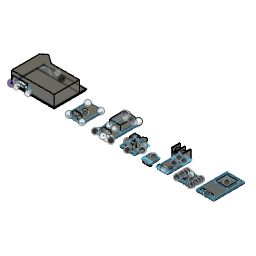
3D Module (Autodesk Fusion 360 design; units mm, degrees)
Autodesk Fusion 360 part; units mm, degrees
note: some values were not read from the file. Set by a fixed rule: which sketch regions a step uses.
sketch "Sketch3" plane through (0, 0, 0) normal (0, 0, 1) x (1, 0, 0)
sketch "LUX" plane through (0, 0, 0) normal (0, 0, 1) x (1, 0, 0)
  line L0 (77.07, 0) -> (94.93, 0)
  line L1 (97, 2.07) -> (97, 27.93)
  line L2 (94.93, 30) -> (77.07, 30)
  line L3 (75, 27.93) -> (75, 2.07)
  line L4 (86, 0) -> (86, 30) construction
  line L5 (86, 0) -> (91, 0) construction
  line L6 (91, 0) -> (91, 6) construction
  line L7 (91, 6) -> (86, 6) construction
  line L8 (86, 6) -> (86, 0) construction
  line L9 (91, 6) -> (81, 6)
  line L10 (81, 6) -> (81, 0)
  line L11 (81, 0) -> (91, 0)
  line L12 (91, 0) -> (91, 6)
  arc A0 (77.07, 30) -> (75, 27.93) centre (77.07, 27.93) ccw
  arc A1 (97, 27.93) -> (94.93, 30) centre (94.93, 27.93) ccw
  arc A2 (75, 2.07) -> (77.07, 0) centre (77.07, 2.07) ccw
  arc A3 (94.93, 0) -> (97, 2.07) centre (94.93, 2.07) ccw
  circle A4 centre (86, 15) radius 2.5
  dimension "d32" = 2.07
  constraint horizontal L0
  constraint vertical L1
  constraint horizontal L2
  constraint vertical L3
  constraint horizontal L5
  constraint vertical L6
  constraint horizontal L7
  constraint vertical L8
  constraint horizontal L9
  constraint vertical L10
  constraint horizontal L11
  constraint vertical L12
  constraint coincident L2 L4.end
  constraint tangent L2 A0
  constraint tangent L3 A0
  constraint tangent L1 A1
  constraint tangent L2 A1
  constraint equal A0 A1
  constraint coincident L0 L4.start
  constraint tangent L3 A2
  constraint tangent L0 A2
  constraint equal A0 A2
  constraint tangent L1 A3
  constraint tangent L0 A3
  constraint equal A0 A3
  constraint midpoint L4 A4.centre
  measures "d32" radius of A0
sketch "DHT" plane through (0, 0, 0) normal (0, 0, 1) x (1, 0, 0)
  line L0 (117.7, 0) -> (134.3, 0)
  line L1 (137, 2.7) -> (137, 38.8)
  line L2 (134.3, 41.5) -> (117.7, 41.5)
  line L3 (115, 38.8) -> (115, 2.7)
  arc A0 (117.7, 41.5) -> (115, 38.8) centre (117.7, 38.8) ccw
  arc A1 (137, 38.8) -> (134.3, 41.5) centre (134.3, 38.8) ccw
  arc A2 (115, 2.7) -> (117.7, 0) centre (117.7, 2.7) ccw
  arc A3 (134.3, 0) -> (137, 2.7) centre (134.3, 2.7) ccw
  line L4 (126, 6) -> (131, 6) construction
  line L5 (131, 0) -> (126, 0) construction
  line L6 (131, 6) -> (121, 6)
  line L7 (121, 6) -> (121, 0)
  line L8 (121, 0) -> (131, 0)
  line L9 (131, 0) -> (131, 6)
  line L10 (126, 41.5) -> (133.5, 41.5) construction
  line L11 (133.5, 16.5) -> (126, 16.5) construction
  line L12 (133.5, 16.5) -> (118.5, 16.5)
  line L13 (118.5, 41.5) -> (133.5, 41.5)
  line L14 (133.5, 16.5) -> (118.5, 16.5)
  line L15 (118.5, 16.5) -> (118.5, 36.5)
  line L16 (118.5, 36.5) -> (133.5, 36.5)
  line L17 (133.5, 36.5) -> (133.5, 16.5)
  line L18 (126, 41.5) -> (126, 36.5) construction
  line L19 (131.25, 36.5) -> (120.75, 36.5) construction
  line L20 (120.75, 41.5) -> (131.25, 41.5) construction
  line L21 (118.5, 36.5) -> (120.75, 41.5)
  line L22 (131.25, 41.5) -> (133.5, 36.5)
  circle A4 centre (126, 39) radius 1.75
  point P0 (115, 0)
  point P1 (137, 0)
  point P2 (115, 41.5)
  point P3 (126, 39)
  dimension "d25" = 22
  dimension "d26" = 41.5
  dimension "d63" = 2.7
  dimension "d65" = 10
  dimension "d66" = 6
  dimension "d68" = 25
  dimension "d69" = 15
  dimension "d70" = 20
  dimension "d71" = 10.5
  dimension "d72" = 3.5
  constraint horizontal L0
  constraint vertical L1
  constraint horizontal L2
  constraint vertical L3
  constraint coincident P2 L3
  constraint coincident P2 L2
  constraint tangent L3 A0
  constraint tangent L2 A0
  constraint tangent L1 A1
  constraint tangent L2 A1
  constraint equal A0 A1
  constraint coincident P0 L3
  constraint coincident P0 L0
  constraint tangent L3 A2
  constraint tangent L0 A2
  constraint equal A0 A2
  constraint coincident P1 L1
  constraint coincident P1 L0
  constraint tangent L1 A3
  constraint tangent L0 A3
  constraint equal A0 A3
  constraint midpoint L2 L10.start
  constraint horizontal L4
  constraint horizontal L5
  constraint horizontal L6
  constraint vertical L7
  constraint horizontal L8
  constraint vertical L9
  constraint horizontal L10
  constraint horizontal L11
  constraint horizontal L12
  constraint horizontal L13
  constraint horizontal L14
  constraint vertical L15
  constraint horizontal L16
  constraint vertical L17
  constraint midpoint L16 L18.end
  constraint horizontal L19
  constraint parallel L19 L20
  constraint midpoint L18 P3
  constraint coincident P3 A4.centre
  measures "d25" distance of P0 P1
  measures "d26" distance of P0 P2
  measures "d63" radius of A0
  measures "d65" distance of L4.end L6.end
  measures "d66" distance of L6 L8
  measures "d68" distance of L10.start L11.end
  measures "d69" distance of L11.start L12.end
  measures "d70" distance of L11.start L16.end
  measures "d71" distance of L20.start L20.end
  measures "d72" diameter of A4
sketch "DSM" plane through (0, 0, 0) normal (0, 0, 1) x (1, 0, 0) in component "DSM"
  line L0 (0, 0) -> (58.5, 0)
  line L1 (58.5, 0) -> (58.5, 35)
  line L2 (58.5, 35) -> (0, 35)
  line L3 (0, 35) -> (0, 0)
  line L4 (0, 0) -> (58.5, 0)
  line L5 (58.5, 0) -> (58.5, 44)
  line L6 (58.5, 44) -> (0, 44)
  line L7 (0, 44) -> (0, 0)
  line L8 (0, 35) -> (19.5, 35) construction
  line L9 (19.5, 44) -> (0, 44) construction
  line L10 (0, 44) -> (0, 35) construction
  line L11 (0, 44) -> (7, 44) construction
  line L12 (7, 0) -> (0, 0) construction
  line L13 (0, 0) -> (0, 44) construction
  line L14 (7, 44) -> (19.5, 35)
  line L15 (7, 44) -> (0, 38.3431)
  line L16 (29.25, 44) -> (29.25, 35) construction
  circle A0 centre (29.25, 39.5) radius 2
  line L17 (5.5, 0) -> (17.5, 0)
  line L18 (17.5, 0) -> (17.5, 5)
  line L19 (17.5, 5) -> (5.5, 5)
  line L20 (5.5, 5) -> (5.5, 0)
  line L21 (0, 0) -> (23, 0)
  line L22 (0, 5) -> (0, 0)
  line L23 (17.5, 5) -> (22, 5)
  line L24 (22, 5) -> (22, 0)
  line L25 (22, 0) -> (17.5, 0) construction
  line L26 (17.5, 0) -> (17.5, 5) construction
  line L27 (5.5, 5) -> (1, 5)
  line L28 (1, 5) -> (1, 0)
  line L29 (1, 0) -> (5.5, 0) construction
  line L30 (5.5, 0) -> (5.5, 5) construction
  dimension "d1" = 58.5
  dimension "d2" = 35
  dimension "d3" = 44
  dimension "d7" = 4
  constraint horizontal L0
  constraint vertical L1
  constraint horizontal L2
  constraint vertical L3
  constraint coincident L0.start L3.end
  constraint horizontal L4
  constraint vertical L5
  constraint horizontal L6
  constraint vertical L7
  constraint horizontal L8
  constraint horizontal L9
  constraint vertical L10
  constraint horizontal L11
  constraint horizontal L12
  constraint vertical L13
  constraint coincident L10 L15.end
  constraint equal L5 L13
  constraint midpoint L6 L16.start
  constraint midpoint L2 L16.end
  constraint midpoint L16 A0.centre
  constraint horizontal L17
  constraint vertical L18
  constraint horizontal L19
  constraint vertical L20
  constraint coincident L12 L17.start
  constraint horizontal L21
  constraint vertical L22
  constraint horizontal L23
  constraint vertical L24
  constraint horizontal L25
  constraint vertical L26
  constraint horizontal L27
  constraint vertical L28
  constraint horizontal L29
  constraint vertical L30
  measures "d1" distance of L0.start L0.end
  measures "d2" distance of L0.start L2.end
  measures "d3" distance of L0.start L6.end
  measures "d7" diameter of A0
extrude "Extrude7" add sketch "DSM" along normal blind 15.5 contours L0 L1 L2 L3 L4 L5 L7 L19 L21 L22 L23 L24 L27 L28 | L0 L4 L20 L21 L27 L28 | L0 L4 L17 L18 L19 L20 L21 | L2 L7 L14 L15 | L0 L4 L18 L21 L23 L24 makes body 1 in component "DSM"
extrude "Extrude4" cut sketch "DSM" along normal blind 10 contours L0 L4 L20 L21 L27 L28 | L0 L4 L17 L18 L19 L20 L21 | L0 L4 L18 L21 L23 L24 bodies 1 in component "DSM"
extrude "Extrude5" add sketch "DSM" against normal blind 1.5 bodies 1 in component "DSM"
extrude "Extrude8" add sketch "DSM" along normal blind 5 separate body contours L0 L4 L17 L18 L19 L20 L21 makes body 2
shell "Shell2" thickness 0.5 removed faces 1 at (9.5, 0, 1.6667) on bodies 2
copy_body "CutPasteBodies1" bodies 2 removing the originals makes body 3 in component "DSM"
extrude "Extrude9" add sketch "LUX" along normal blind 3 separate body contours A4 makes body 4
extrude "Extrude11" add sketch "LUX" against normal blind 1 contours L0 L1 L2 L3 L9 L10 L12 A0 A1 A2 A3 | L0 L9 L10 L11 L12 | A4 bodies 4
copy_body "Body->Comp1" bodies 4 removing the originals makes body 5 in component "LUX"
extrude "Extrude12" add sketch "LUX" along normal blind 5.5 separate body contours L0 L9 L10 L11 L12 makes body 6
shell "Shell4" thickness 0.5 removed faces 1 at (84.3333, 0, 3.6667) on bodies 6
copy_body "CutPasteBodies1'" bodies 6 removing the originals makes body 7 in component "LUX"
extrude "Extrude13" add sketch "DHT" along normal blind 8 separate body contours L12 L14 L15 L16 L17 makes body 8
extrude "Extrude14" add sketch "DHT" along normal blind 1.5 contours L2 L13 L16 L21 L22 bodies 8
extrude "Extrude15" add sketch "DHT" against normal blind 1 contours L0 L1 L2 L3 A0 A1 A2 A3 L6 L7 L9 L12 L13 L14 L15 L17 L21 L22 | L0 L6 L7 L8 L9 bodies 8
copy_body "Body->Comp2" bodies 8 removing the originals makes body 9 in component "DHT22"
extrude "Extrude16" add sketch "DHT" along normal blind 5.5 separate body contours L0 L6 L7 L8 L9 makes body 10
shell "Shell5" thickness 0.5 removed faces 1 at (124.3333, 0, 3.6667) on bodies 10
copy_body "CutPasteBodies1''" bodies 10 removing the originals makes body 11 in component "DHT22"
sketch "WSP" plane through (0, 0, 0) normal (0, 0, 1) x (1, 0, 0)
  line L0 (150, 0) -> (170, 0)
  line L1 (170, 0) -> (170, 20)
  line L2 (170, 20) -> (150, 20)
  line L3 (150, 20) -> (150, 0)
  line L4 (160, 20) -> (160, 0) construction
  circle A0 centre (150, 10) radius 2
  circle A1 centre (170, 10) radius 2
  circle A2 centre (160, 20) radius 2
  circle A3 centre (160, 0) radius 2
  circle A4 centre (150, 10) radius 1
  circle A5 centre (170, 10) radius 1
  line L5 (160, 2) -> (165, 2) construction
  line L6 (165, 2) -> (165, 7) construction
  line L7 (165, 7) -> (160, 7) construction
  line L8 (160, 7) -> (160, 2) construction
  line L9 (165, 7) -> (155, 7)
  line L10 (155, 7) -> (155, 2)
  line L11 (155, 2) -> (165, 2)
  line L12 (165, 2) -> (165, 7)
  line L13 (150, 20) -> (157, 20)
  line L14 (157, 20) -> (157, 13)
  line L15 (157, 13) -> (150, 13)
  line L16 (150, 13) -> (150, 20)
  circle A6 centre (166, 16) radius 4
  dimension "d82" = 20
  dimension "d83" = 20
  dimension "d84" = 4
  dimension "d85" = 4
  dimension "d86" = 4
  dimension "d87" = 4
  dimension "d88" = 2
  dimension "d89" = 2
  dimension "d91" = 5
  dimension "d92" = 10
  dimension "d93" = 7
  dimension "d94" = 7
  dimension "d95" = 4
  constraint horizontal L0
  constraint vertical L1
  constraint horizontal L2
  constraint vertical L3
  constraint midpoint L2 L4.start
  constraint midpoint L0 L4.end
  constraint midpoint L3 A0.centre
  constraint midpoint L1 A1.centre
  constraint coincident L4.start A2.centre
  constraint coincident L4.end A3.centre
  constraint concentric A0 A4
  constraint concentric A1 A5
  constraint horizontal L5
  constraint vertical L6
  constraint horizontal L7
  constraint vertical L8
  constraint coincident A3 L5.start
  constraint coincident L4 L5.start
  constraint horizontal L9
  constraint vertical L10
  constraint horizontal L11
  constraint vertical L12
  constraint horizontal L13
  constraint vertical L14
  constraint horizontal L15
  constraint vertical L16
  constraint tangent L2 A6
  constraint tangent L1 A6
  measures "d82" distance of L0.start L0.end
  measures "d83" distance of L0.start L2.end
  measures "d84" diameter of A0
  measures "d85" diameter of A1
  measures "d86" diameter of A2
  measures "d87" diameter of A3
  measures "d88" diameter of A4
  measures "d89" diameter of A5
  measures "d91" distance of L5.start L7.end
  measures "d92" distance of L6.end L9.end
  measures "d93" distance of L2.end L13.end
  measures "d94" distance of L2.end L15.end
  measures "d95" radius of A6
extrude "Extrude17" add sketch "WSP" along normal blind 5 separate body contours L2 L3 L13 L14 L15 L16 makes body 12
extrude "Extrude18" add sketch "WSP" along normal blind 7.5 separate body contours A6 makes body 13
extrude "Extrude19" add sketch "WSP" against normal blind 1.5 contours L9 L10 L11 L12 | L0 L1 L2 L3 A0 A1 A2 A3 L14 L15 A6 | L1 A1 A5 | L1 A1 A5 | L3 A0 A4 | L3 A0 A4 bodies 12 13
copy_body "Body->Comp3" bodies 12 removing the originals makes body 14 in component "WSP_bdy"
extrude "Extrude20" add sketch "WSP" along normal blind 8 separate body contours L9 L10 L11 L12 makes body 15
shell "Shell6" thickness 0.5 removed faces 1 at (160, 5.3333, 8) on bodies 15
copy_body "CutPasteBodies1'''" bodies 15 removing the originals makes body 16 in component "WSP_bdy"
sketch "SGP30" plane through (0, 0, 0) normal (0, 0, 1) x (1, 0, 0)
  line L0 (180, 0) -> (192, 0)
  line L1 (192, 0) -> (192, 12)
  line L2 (192, 12) -> (180, 12)
  line L3 (180, 12) -> (180, 0)
  line L4 (186, 12) -> (186, 0) construction
  line L5 (187.25, 8.7246) -> (184.75, 8.7246)
  line L6 (184.75, 8.7246) -> (184.75, 11.2246)
  line L7 (184.75, 11.2246) -> (187.25, 11.2246)
  line L8 (187.25, 11.2246) -> (187.25, 8.7246)
  line L9 (187.25, 8.7246) -> (184.75, 11.2246) construction
  line L10 (184.75, 8.7246) -> (187.25, 11.2246) construction
  line L11 (186, 0) -> (191, 0) construction
  line L12 (191, 0) -> (191, 2.45) construction
  line L13 (191, 2.45) -> (186, 2.45) construction
  line L14 (186, 2.45) -> (186, 0) construction
  line L15 (191, 2.45) -> (181, 2.45)
  line L16 (181, 2.45) -> (181, 0)
  line L17 (181, 0) -> (191, 0)
  line L18 (191, 0) -> (191, 2.45)
  point P0 (186, 9.9746)
  dimension "d105" = 12
  dimension "d106" = 12
  dimension "d107" = 2.5
  dimension "d108" = 2.5
  dimension "d110" = 2.45
  dimension "d111" = 10
  constraint horizontal L0
  constraint vertical L1
  constraint horizontal L2
  constraint vertical L3
  constraint midpoint L2 L4.start
  constraint midpoint L0 L4.end
  constraint horizontal L5
  constraint perpendicular L5 L6
  constraint parallel L5 L7
  constraint parallel L6 L8
  constraint coincident L9 P0
  constraint coincident L10 P0
  constraint coincident L4 P0
  constraint horizontal L11
  constraint vertical L12
  constraint horizontal L13
  constraint vertical L14
  constraint horizontal L15
  constraint vertical L16
  constraint horizontal L17
  constraint vertical L18
  measures "d105" distance of L0.start L0.end
  measures "d106" distance of L0.start L2.end
  measures "d107" distance of L6.end L7.end
  measures "d108" distance of L5.end L6.end
  measures "d110" distance of L4.end L13.end
  measures "d111" distance of L12.end L15.end
extrude "Extrude21" add sketch "SGP30" along normal blind 1 separate body contours L5 L6 L7 L8 makes body 17
extrude "Extrude22" add sketch "SGP30" against normal blind 1.5 contours L0 L1 L2 L3 L15 L16 L18 | L0 L15 L16 L17 L18 | L5 L6 L7 L8 bodies 17
extrude "Extrude23" add sketch "SGP30" against normal blind 4.5 contours L0 L15 L16 L17 L18 bodies 17
copy_body "Body->Comp4" bodies 17 removing the originals makes body 18 in component "SGP30"
sketch "Thermo" plane through (0, 0, 0) normal (0, 0, 1) x (1, 0, 0)
  line L0 (200, 0) -> (215.5, 0)
  line L1 (215.5, 0) -> (215.5, 32)
  line L2 (215.5, 32) -> (200, 32)
  line L3 (200, 32) -> (200, 0)
  line L4 (200, 32) -> (215.5, 32)
  line L5 (215.5, 32) -> (215.5, 21)
  line L6 (215.5, 21) -> (200, 21)
  line L7 (200, 21) -> (200, 32)
  line L8 (208.25, 32) -> (207.25, 32)
  line L9 (207.25, 32) -> (207.25, 21)
  line L10 (207.25, 21) -> (208.25, 21)
  line L11 (208.25, 21) -> (208.25, 32)
  line L12 (200, 32) -> (201, 32)
  line L13 (201, 32) -> (201, 21)
  line L14 (201, 21) -> (200, 21)
  line L15 (200, 21) -> (200, 32)
  line L16 (215.5, 32) -> (214.5, 32)
  line L17 (214.5, 32) -> (214.5, 21)
  line L18 (214.5, 21) -> (215.5, 21)
  line L19 (215.5, 21) -> (215.5, 32)
  line L20 (215.5, 26.5) -> (200, 26.5) construction
  circle A0 centre (204.125, 26.5) radius 3.125
  circle A1 centre (211.375, 26.5) radius 3.125
  line L21 (207.25, 23.375) -> (201, 23.375)
  line L22 (201, 23.375) -> (201, 29.625) construction
  line L23 (201, 29.625) -> (207.25, 29.625)
  line L24 (207.25, 29.625) -> (207.25, 23.375) construction
  line L25 (214.5, 23.375) -> (208.25, 23.375)
  line L26 (208.25, 23.375) -> (208.25, 29.625)
  line L27 (208.25, 29.625) -> (214.5, 29.625)
  line L28 (214.5, 29.625) -> (214.5, 23.375)
  line L29 (207.75, 0) -> (207.75, 32) construction
  circle A2 centre (207.75, 16) radius 2
  line L30 (207.75, 0) -> (214, 0)
  line L31 (214, 0) -> (214, 2.5)
  line L32 (214, 2.5) -> (207.75, 2.5)
  line L33 (214, 2.5) -> (201.5, 2.5)
  line L34 (201.5, 2.5) -> (201.5, 0)
  line L35 (201.5, 0) -> (214, 0)
  line L36 (214, 0) -> (214, 2.5)
  line L37 (214, 5.5) -> (210, 5.5)
  line L38 (210, 5.5) -> (210, 10.5)
  line L39 (210, 10.5) -> (214, 10.5)
  line L40 (214, 10.5) -> (214, 5.5)
  point P0 (207.75, 26.5)
  point P1 (204.125, 26.5)
  point P2 (211.375, 26.5)
  point P3 (212, 8)
  dimension "d118" = 15.5
  dimension "d119" = 32
  dimension "d120" = 11
  dimension "d121" = 1
  dimension "d123" = 1
  dimension "d124" = 1
  dimension "d125" = 6.25
  dimension "d126" = 6.25
  dimension "d127" = 6.25
  dimension "d128" = 6.25
  dimension "d129" = 4
  dimension "d131" = 2.5
  dimension "d132" = 12.5
  dimension "d133" = 4
  dimension "d134" = 5
  constraint horizontal L0
  constraint vertical L1
  constraint horizontal L2
  constraint vertical L3
  constraint horizontal L4
  constraint vertical L5
  constraint horizontal L6
  constraint vertical L7
  constraint horizontal L8
  constraint perpendicular L8 L9
  constraint parallel L8 L10
  constraint parallel L9 L11
  constraint horizontal L12
  constraint vertical L13
  constraint horizontal L14
  constraint vertical L15
  constraint coincident L6 L13.end
  constraint horizontal L16
  constraint vertical L17
  constraint horizontal L18
  constraint vertical L19
  constraint midpoint L19 L20.start
  constraint midpoint L7 L20.end
  constraint perpendicular L3 L20
  constraint tangent L13 A0
  constraint tangent L17 A1
  constraint horizontal L21
  constraint perpendicular L21 L22
  constraint parallel L21 L23
  constraint parallel L22 L24
  constraint coincident P1 A0.centre
  constraint horizontal L25
  constraint perpendicular L25 L26
  constraint parallel L25 L27
  constraint parallel L26 L28
  constraint coincident P2 A1.centre
  constraint midpoint L0 L29.start
  constraint midpoint L2 L29.end
  constraint midpoint L29 A2.centre
  constraint horizontal L30
  constraint vertical L31
  constraint horizontal L32
  constraint horizontal L33
  constraint vertical L34
  constraint horizontal L35
  constraint vertical L36
  constraint horizontal L37
  constraint perpendicular L37 L38
  constraint parallel L37 L39
  constraint parallel L38 L40
  measures "d118" distance of L0.start L0.end
  measures "d119" distance of L0.start L2.end
  measures "d120" distance of L2.end L6.end
  measures "d121" distance of L9.end L10.end
  measures "d123" distance of L2.end L12.end
  measures "d124" distance of L1.end L16.end
  measures "d125" distance of L22.end L23.end
  measures "d126" distance of L21.end L22.end
  measures "d127" distance of L26.end L27.end
  measures "d128" distance of L25.end L26.end
  measures "d129" diameter of A2
  measures "d131" distance of L29.start L32.end
  measures "d132" distance of L31.end L33.end
  measures "d133" distance of L38.end L39.end
  measures "d134" distance of L37.end L38.end
extrude "Extrude24" add sketch "Thermo" along normal blind 7 separate body contours L2 L3 L4 L6 L7 L12 L13 L14 L15 | L6 L9 L13 L21 | L2 L4 L9 L13 L23 | L2 L4 L6 L8 L9 L10 L11 L26 | L13 A0 L21 | L13 A0 L23 | L6 L11 L17 L25 | L9 A0 L21 | A0 | L1 L2 L4 L5 L6 L16 L17 L18 L19 L28 | L2 L4 L11 L17 L27 | L9 A0 L23 | L11 A1 L25 L26 | L11 A1 L26 L27 | L17 A1 L25 L28 | A1 | L17 A1 L27 L28 makes body 19
extrude "Extrude25" add sketch "Thermo" along normal blind 12.5 contours L2 L3 L4 L6 L7 L12 L13 L14 L15 | L2 L4 L6 L8 L9 L10 L11 L26 | L1 L2 L4 L5 L6 L16 L17 L18 L19 L28 bodies 19
extrude "Extrude26" add sketch "Thermo" along normal blind 8 contours L13 A0 L21 | L13 A0 L23 | L9 A0 L21 | A0 | L9 A0 L23 | L11 A1 L25 L26 | L11 A1 L26 L27 | L17 A1 L25 L28 | A1 | L17 A1 L27 L28 bodies 19
extrude "Extrude27" add sketch "Thermo" along normal blind 10 contours A0 | A1 bodies 19
extrude "Extrude28" add sketch "Thermo" along normal blind 2 separate body contours L37 L38 L39 L40 makes body 20
extrude "Extrude29" add sketch "Thermo" along normal blind 2.5 separate body contours L0 L30 L31 L32 L33 L34 L35 L36 makes body 21
extrude "Extrude30" add sketch "Thermo" against normal blind 1.5 contours L0 L1 L3 L6 L10 L14 L18 L31 L32 L33 L34 L36 | L0 L30 L31 L32 L33 L34 L35 L36 | L2 L3 L4 L6 L7 L12 L13 L14 L15 | L6 L9 L13 L21 | L2 L4 L9 L13 L23 | L2 L4 L6 L8 L9 L10 L11 L26 | L13 A0 L21 | L13 A0 L23 | L6 L11 L17 L25 | L9 A0 L21 | A0 | L1 L2 L4 L5 L6 L16 L17 L18 L19 L28 | L2 L4 L11 L17 L27 | L9 A0 L23 | L11 A1 L25 L26 | L11 A1 L26 L27 | L17 A1 L25 L28 | A1 | L17 A1 L27 L28 | L37 L38 L39 L40 bodies 20 19 21
sketch "Busk_mini" plane through (0, 0, 0) normal (0, 0, 1) x (1, 0, 0)
  line L0 (225, 0) -> (247, 0)
  line L1 (247, 0) -> (247, 17)
  line L2 (247, 17) -> (225, 17)
  line L3 (225, 17) -> (225, 0)
  line L4 (247, 17) -> (243.5, 17)
  line L5 (243.5, 17) -> (243.5, 0) construction
  line L6 (243.5, 0) -> (247, 0)
  line L7 (247, 0) -> (247, 17)
  line L8 (225, 17) -> (228.5, 17)
  line L9 (228.5, 17) -> (228.5, 0) construction
  line L10 (228.5, 0) -> (225, 0)
  line L11 (225, 0) -> (225, 17)
  line L12 (225, 17) -> (247, 17) construction
  line L13 (247, 17) -> (247, 11) construction
  line L14 (247, 11) -> (225, 11) construction
  line L15 (225, 11) -> (225, 17) construction
  line L16 (225, 0) -> (247, 0) construction
  line L17 (247, 0) -> (247, 6) construction
  line L18 (247, 6) -> (225, 6) construction
  line L19 (225, 6) -> (225, 0) construction
  line L20 (243.5, 17) -> (247, 17) construction
  line L21 (247, 17) -> (247, 11) construction
  line L22 (247, 11) -> (243.5, 11) construction
  line L23 (243.5, 11) -> (243.5, 17) construction
  line L24 (243.5, 17) -> (247, 17)
  line L25 (247, 17) -> (247, 11)
  line L26 (247, 11) -> (243.5, 11)
  line L27 (243.5, 11) -> (243.5, 17)
  line L28 (225, 17) -> (228.5, 17)
  line L29 (228.5, 17) -> (228.5, 11)
  line L30 (228.5, 11) -> (225, 11)
  line L31 (225, 11) -> (225, 17)
  line L32 (228.5, 6) -> (225, 6)
  line L33 (225, 6) -> (225, 0)
  line L34 (225, 0) -> (228.5, 0)
  line L35 (228.5, 0) -> (228.5, 6)
  line L36 (243.5, 6) -> (247, 6)
  line L37 (247, 6) -> (247, 0)
  line L38 (247, 0) -> (243.5, 0)
  line L39 (243.5, 0) -> (243.5, 6)
  line L40 (225, 14) -> (228.5, 14) construction
  line L41 (243.5, 14) -> (247, 14) construction
  line L42 (243.5, 3) -> (247, 3) construction
  line L43 (228.5, 3) -> (225, 3) construction
  line L44 (225, 17) -> (228.5, 17) construction
  line L45 (228.5, 17) -> (228.5, 14) construction
  line L46 (228.5, 14) -> (225, 14) construction
  line L47 (225, 14) -> (225, 17) construction
  line L48 (225, 15.5) -> (247, 15.5) construction
  line L49 (225, 14) -> (228.5, 14) construction
  line L50 (228.5, 14) -> (228.5, 11) construction
  line L51 (228.5, 11) -> (225, 11) construction
  line L52 (225, 11) -> (225, 14) construction
  line L53 (226.75, 17) -> (226.75, 0) construction
  line L54 (245.25, 17) -> (245.25, 0) construction
  circle A0 centre (226.75, 15.5) radius 0.5
  circle A1 centre (226.75, 12.5) radius 0.5
  circle A2 centre (245.25, 15.5) radius 0.5
  circle A3 centre (245.25, 12.5) radius 0.5
  line L55 (225, 6) -> (228.5, 6)
  line L56 (228.5, 6) -> (228.5, 3)
  line L57 (228.5, 3) -> (225, 3)
  line L58 (225, 3) -> (225, 6)
  line L59 (225, 3) -> (228.5, 3)
  line L60 (228.5, 3) -> (228.5, 0)
  line L61 (228.5, 0) -> (225, 0)
  line L62 (225, 0) -> (225, 3)
  circle A4 centre (226.75, 4.5) radius 0.5
  circle A5 centre (226.75, 1.5) radius 0.5
  circle A6 centre (245.25, 1.5) radius 0.5
  circle A7 centre (245.25, 4.5) radius 0.5
  line L63 (246.25, 10) -> (244.25, 10)
  line L64 (244.25, 10) -> (244.25, 7)
  line L65 (244.25, 7) -> (246.25, 7)
  line L66 (246.25, 7) -> (246.25, 10)
  line L67 (227.75, 7) -> (225.75, 7)
  line L68 (225.75, 7) -> (225.75, 10)
  line L69 (225.75, 10) -> (227.75, 10)
  line L70 (227.75, 10) -> (227.75, 7)
  line L71 (230, 2) -> (237, 2)
  line L72 (237, 2) -> (237, 9)
  line L73 (237, 9) -> (230, 9)
  line L74 (230, 9) -> (230, 2)
  circle A8 centre (233.1143, 14) radius 1.5
  line L75 (242.4307, 6.75) -> (237.4307, 6.75)
  line L76 (237.4307, 6.75) -> (237.4307, 10.25)
  line L77 (237.4307, 10.25) -> (242.4307, 10.25)
  line L78 (242.4307, 10.25) -> (242.4307, 6.75)
  point P0 (245.25, 8.5)
  point P1 (226.75, 8.5)
  point P2 (239.9307, 8.5)
  dimension "d149" = 22
  dimension "d150" = 17
  dimension "d151" = 3.5
  dimension "d152" = 3.5
  dimension "d153" = 6
  dimension "d154" = 6
  dimension "d156" = 1
  dimension "d157" = 1
  dimension "d158" = 1
  dimension "d159" = 1
  dimension "d160" = 1
  dimension "d161" = 1
  dimension "d162" = 1
  dimension "d163" = 1
  dimension "d168" = 7
  dimension "d169" = 7
  dimension "d170" = 3
  constraint horizontal L0
  constraint vertical L1
  constraint horizontal L2
  constraint vertical L3
  constraint horizontal L4
  constraint vertical L5
  constraint horizontal L6
  constraint vertical L7
  constraint horizontal L8
  constraint vertical L9
  constraint horizontal L10
  constraint vertical L11
  constraint horizontal L12
  constraint vertical L13
  constraint horizontal L14
  constraint vertical L15
  constraint horizontal L16
  constraint vertical L17
  constraint horizontal L18
  constraint vertical L19
  constraint horizontal L20
  constraint vertical L21
  constraint horizontal L22
  constraint vertical L23
  constraint horizontal L24
  constraint vertical L25
  constraint horizontal L26
  constraint vertical L27
  constraint horizontal L28
  constraint vertical L29
  constraint horizontal L30
  constraint vertical L31
  constraint coincident L9 L29.end
  constraint coincident L14 L29.end
  constraint horizontal L32
  constraint vertical L33
  constraint horizontal L34
  constraint vertical L35
  constraint coincident L18 L32.start
  constraint coincident L9 L32.start
  constraint horizontal L36
  constraint vertical L37
  constraint horizontal L38
  constraint vertical L39
  constraint coincident L7 L0.end
  constraint coincident L17 L0.end
  constraint coincident L5 L36.start
  constraint coincident L18 L36.start
  constraint midpoint L31 L40.start
  constraint midpoint L29 L40.end
  constraint midpoint L27 L41.start
  constraint midpoint L21 L41.end
  constraint midpoint L39 L42.start
  constraint midpoint L17 L42.end
  constraint perpendicular L1 L42
  constraint midpoint L35 L43.start
  constraint midpoint L19 L43.end
  constraint horizontal L44
  constraint vertical L45
  constraint horizontal L46
  constraint vertical L47
  constraint horizontal L48
  constraint midpoint L47 L48.start
  constraint coincident L1 L48.end
  constraint coincident L25 L48.end
  constraint horizontal L49
  constraint vertical L50
  constraint horizontal L51
  constraint vertical L52
  constraint midpoint L44 L53.start
  constraint midpoint L34 L53.end
  constraint midpoint L20 L54.start
  constraint midpoint L38 L54.end
  constraint coincident L53 A0.centre
  constraint coincident L48 A0.centre
  constraint coincident L53 A1.centre
  constraint coincident L54 A2.centre
  constraint coincident L48 A2.centre
  constraint coincident L54 A3.centre
  constraint horizontal L55
  constraint vertical L56
  constraint horizontal L57
  constraint vertical L58
  constraint horizontal L59
  constraint vertical L60
  constraint horizontal L61
  constraint vertical L62
  constraint coincident L53 A4.centre
  constraint coincident L53 A5.centre
  constraint coincident L54 A6.centre
  constraint coincident L54 A7.centre
  constraint horizontal L63
  constraint perpendicular L63 L64
  constraint parallel L63 L65
  constraint parallel L64 L66
  constraint midpoint L54 P0
  constraint horizontal L67
  constraint perpendicular L67 L68
  constraint parallel L67 L69
  constraint parallel L68 L70
  constraint midpoint L53 P1
  constraint horizontal L71
  constraint vertical L72
  constraint horizontal L73
  constraint vertical L74
  constraint horizontal L75
  constraint perpendicular L75 L76
  constraint parallel L75 L77
  constraint parallel L76 L78
  measures "d149" distance of L0.start L0.end
  measures "d150" distance of L0.start L2.end
  measures "d151" distance of L1.end L4.end
  measures "d152" distance of L2.end L8.end
  measures "d153" distance of L2.end L14.end
  measures "d154" distance of L0.start L18.end
  measures "d156" diameter of A0
  measures "d157" diameter of A1
  measures "d158" diameter of A2
  measures "d159" diameter of A3
  measures "d160" diameter of A4
  measures "d161" diameter of A5
  measures "d162" diameter of A6
  measures "d163" diameter of A7
  measures "d168" distance of L71.start L71.end
  measures "d169" distance of L71.start L73.end
  measures "d170" diameter of A8
extrude "Extrude31" add sketch "Busk_mini" along normal blind 2.7 separate body contours L71 L72 L73 L74 makes body 22
extrude "Extrude32" add sketch "Busk_mini" along normal blind 2 separate body contours L75 L76 L77 L78 makes body 23
extrude "Extrude33" add sketch "Busk_mini" along normal blind 1 separate body contours A8 makes body 24
extrude "Extrude34" add sketch "Busk_mini" along normal blind 1 separate body contours L63 L64 L65 L66 | L67 L68 L69 L70 makes body 25 at (226.4167, 9, 0) makes body 26 at (244.9167, 9, 0)
extrude "Extrude35" add sketch "Busk_mini" against normal blind 1.5 contours L0 L3 L10 L11 L33 L34 L35 L57 L59 L60 L61 L62 | L0 L1 L2 L3 L7 L11 L26 L27 L29 L30 L32 L35 L36 L39 L55 L56 L60 | L3 L11 L32 L33 L35 L55 L56 L57 L58 L59 | L0 L1 L6 L7 L36 L37 L38 L39 | L2 L3 L8 L11 L28 L29 L30 L31 | L1 L2 L4 L7 L24 L25 L26 L27 | L63 L64 L65 L66 | L67 L68 L69 L70 | L71 L72 L73 L74 | A8 | L75 L76 L77 L78 bodies 22 23 24 25 26
sketch "SD Shield" plane through (0, 0, 0) normal (0, 0, 1) x (1, 0, 0)
  line L0 (255, 0) -> (279, 0)
  line L1 (279, 0) -> (279, 42)
  line L2 (279, 42) -> (255, 42)
  line L3 (255, 42) -> (255, 0)
  line L4 (274.5, 22.6115) -> (259.5, 22.6115)
  line L5 (259.5, 22.6115) -> (259.5, 37.6115)
  line L6 (259.5, 37.6115) -> (274.5, 37.6115)
  line L7 (274.5, 37.6115) -> (274.5, 22.6115)
  line L8 (274.5, 3.7012) -> (259.5, 3.7012)
  line L9 (259.5, 3.7012) -> (259.5, 1.2012)
  line L10 (259.5, 1.2012) -> (274.5, 1.2012)
  line L11 (274.5, 1.2012) -> (274.5, 3.7012)
  point P0 (267, 30.1115)
  point P1 (267, 2.4512)
  dimension "d183" = 24
  dimension "d184" = 42
  dimension "d185" = 15
  dimension "d186" = 15
  dimension "d187" = 15
  dimension "d188" = 2.5
  constraint horizontal L0
  constraint vertical L1
  constraint horizontal L2
  constraint vertical L3
  constraint horizontal L4
  constraint perpendicular L4 L5
  constraint parallel L4 L6
  constraint parallel L5 L7
  constraint horizontal L8
  constraint perpendicular L8 L9
  constraint parallel L8 L10
  constraint parallel L9 L11
  measures "d183" distance of L0.start L0.end
  measures "d184" distance of L0.start L2.end
  measures "d185" distance of L5.end L6.end
  measures "d186" distance of L4.end L5.end
  measures "d187" distance of L9.end L10.end
  measures "d188" distance of L8.end L9.end
extrude "Extrude36" add sketch "SD Shield" along normal blind 1.5 separate body contours L4 L5 L6 L7 makes body 27
extrude "Extrude37" add sketch "SD Shield" along normal blind 2.5 separate body contours L8 L9 L10 L11 makes body 28
extrude "Extrude38" add sketch "SD Shield" against normal blind 1.5 contours L0 L1 L2 L3 | L4 L5 L6 L7 | L8 L9 L10 L11 bodies 27 28
component "DSM" placed x (1, 0, 0) y (0, 1, 0) z (0, 0, 1) at (0, 0, 0)
component "LUX" placed x (1, 0, 0) y (0, 1, 0) z (0, 0, 1) at (0, 0, 0)
component "DHT22" placed x (1, 0, 0) y (0, 1, 0) z (0, 0, 1) at (0, 0, 0)
component "WSP_bdy" placed x (1, 0, 0) y (0, 1, 0) z (0, 0, 1) at (0, 0, 0)
component "SGP30" placed x (1, 0, 0) y (0, 1, 0) z (0, 0, 1) at (0, 0, 0)
equation "d44 = 17 mm - 1.5 mm"
equation "d98 = 9 mm - 1.5 mm"
equation "d102 = 9.5 mm - 1.5 mm"
equation "d112 = 2.5 mm - 1.5 mm"
equation "d135 = 8.5 mm - 1.5 mm"
equation "d137 = 14 mm - 1.5 mm"
equation "d173 = 4.2 mm - 1.5 mm"
equation "d175 = 3.5 mm - 1.5 mm"
named bodies: "DSM", "DSM_con", "LUX_bdy", "LUX_con", "DHT", "DHT_con", "WSP_bdy", "WSP_con", "SGP30", "Thermo", "Buck Mini", "SD Shield"
